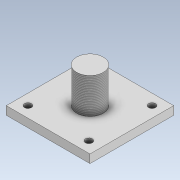
# Autodesk Inventor part: conector cardan
Saved by Autodesk Inventor 2021 (Build 250183000, 183)
## iProperties
Created: 2021-04-23
Part Number: conector cardan
Material: Genérico
Document SubType Name: Modeling
Designer: equip
Density: 1 g/cm^3
Appearance: Valor por defecto
Author: equip
Autodesk Inventor part; units mm, degrees
ref_plane "YZ Plane" through (0, 0, 0) normal (1, 0, 0) x (0, 1, 0)
ref_plane "XZ Plane" through (0, 0, 0) normal (0, 1, 0) x (-1, 0, 0)
ref_plane "XY Plane" through (0, 0, 0) normal (0, 0, 1) x (1, 0, 0)
sketch "Boceto1" plane through (0, 0, 0) normal (0, 1, 0) x (-1, 0, 0)
  circle A0 centre (0, 0) radius 19.05
  line L0 (0, 0) -> (0, 22.5) construction
  line L1 (0, 22.5) -> (-32.5, 22.5) construction
  line L2 (-32.5, 22.5) -> (32.5, 22.5)
  line L3 (32.5, 22.5) -> (32.5, -22.5)
  line L4 (32.5, -22.5) -> (-32.5, -22.5)
  line L5 (-32.5, -22.5) -> (-32.5, 22.5)
  dimension "d0" = 38.1
  dimension "d1" = 22.5
  dimension "d2" = 32.5
  dimension "d3" = 65
  dimension "d4" = 45
  constraints: 12 end point, 2 parallel, 2 perpendicular, 1 centre point, 1 coincident, 1 horizontal, 1 vertical
  measures "d0" diameter of A0
  measures "d1" distance of L0.start L0.end
  measures "d2" distance of L0.end L1.end
  measures "d3" distance of L3.end L4.end
  measures "d4" distance of L2.end L3.end
extrude "Extrusión1" add sketch "Boceto1" along normal blind 50.8 contours A0
sketch "Boceto2" plane through (0, 0, 0) normal (0, -1, 0) x (1, 0, 0)
  line L0 (0, 0) -> (-60, 0) construction
  line L1 (-60, 0) -> (-60, -60) construction
  line L2 (-60, -60) -> (60, -60)
  line L3 (60, -60) -> (60, 60)
  line L4 (60, 60) -> (-60, 60)
  line L5 (-60, 60) -> (-60, -60)
  dimension "d7" = 60
  dimension "d8" = 60
  dimension "d9" = 120
  dimension "d10" = 120
  constraints: 12 end point, 2 horizontal, 2 parallel, 2 perpendicular
  measures "d7" distance of L0.start L0.end
  measures "d8" distance of L0.end L1.end
  measures "d9" distance of L4.end L3.end
  measures "d10" distance of L3.end L2.end
extrude "Extrusión2" add sketch "Boceto2" along normal blind 12
thread "Rosca1" size "M16x2" class "6g" standard "ANSI Metric M Profile" full length
sketch "Sketch4" plane through (0, 0, 0) normal (0, 1, 0) x (1, 0, 0)
  line L0 (60, 60) -> (60, -60) construction
  line L1 (-60, 60) -> (60, 60) construction
  line L2 (-60, -60) -> (-60, 60) construction
  line L3 (60, -60) -> (-60, -60) construction
  circle A0 centre (0, 0) radius 19.05 construction
  line L4 (-60, 60) -> (60, 60) construction
  line L5 (0, 60) -> (0, -60) construction
  line L6 (60, 60) -> (60, -60) construction
  line L7 (60, 0) -> (-60, 0) construction
  point P0 (-44.5, 44.5)
  point P1 (44.5, 44.5)
  point P2 (-44.5, -44.5)
  point P3 (42.8657, -44.5)
  dimension "d34" = 89
  dimension "d35" = 89
  dimension "d36" = 89
  constraints: 4 end point, 4 midpoint, 2 symmetric about line
  measures "d34" distance of point (44.5, 44.5) point (-44.5, 44.5)
  measures "d35" distance of point (-44.5, 44.5) point (-44.5, -44.5)
  measures "d36" vertical distance of point (44.5, 44.5) point (42.866, -44.5)
hole "Hole1" at (-44.5, 0, -44.5) at (44.5, 0, -44.5) at (-44.5, 0, 44.5) at (42.8657, 0, 44.5) direction (0, -1, 0) diameter 10 end through all
equation "\"d7\" = 0.5 * d9"
equation "\"d8\" = 0.5 * d10"
